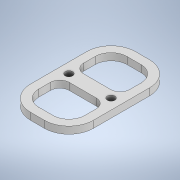
# Autodesk Inventor part: Top Seal 1
Saved by Autodesk Inventor 2021 (Build 250183000, 183)
## iProperties
Created: 2020-06-01
Part Number: Top Seal 1
Material: Generic
Document SubType Name: Modeling
Designer: jgray
Density: 1 g/cm^3
Appearance: Default
Author: jgray
Autodesk Inventor part; units mm, degrees
ref_plane "YZ Plane" through (0, 0, 0) normal (1, 0, 0) x (0, 1, 0)
ref_plane "XZ Plane" through (0, 0, 0) normal (0, 1, 0) x (-1, 0, 0)
ref_plane "XY Plane" through (0, 0, 0) normal (0, 0, 1) x (1, 0, 0)
sketch "Sketch2" plane through (0, 0, 0) normal (0, 1, 0) x (-1, 0, 0)
  arc A0 (3.5, 8.5) -> (1.5, 10.5) centre (1.5, 8.5) ccw
  arc A1 (1.5, -5.5) -> (3.5, -3.5) centre (1.5, -3.5) ccw
  line L0 (1.5, -5.5) -> (-1.5, -5.5)
  arc A2 (-3.5, -3.5) -> (-1.5, -5.5) centre (-1.5, -3.5) ccw
  arc A3 (-1.5, 10.5) -> (-3.5, 8.5) centre (-1.5, 8.5) ccw
  circle A4 centre (-9.4, -30.5) radius 1.7
  circle A5 centre (9.4, -15) radius 1.7
  circle A6 centre (9.4, 30.5) radius 1.7
  circle A7 centre (-9.4, 30.5) radius 1.7
  circle A8 centre (-9.4, 15) radius 1.7
  circle A9 centre (9.4, 15) radius 1.7
  circle A10 centre (-9.4, -15) radius 1.7
  circle A11 centre (9.4, -30.5) radius 1.7
  line L1 (-13.9, -33.875) -> (-13.9, 33.875)
  line L2 (13.9, -33.875) -> (-13.9, -33.875)
  line L3 (13.9, 33.875) -> (13.9, -33.875)
  line L4 (-13.9, 33.875) -> (13.9, 33.875)
  arc A12 (4.5, 8.5) -> (3.8682, 10.3417) centre (1.5, 8.5) ccw
  line L5 (-1.5, 10.5) -> (1.5, 10.5)
  arc A13 (-4.5, -3.5) -> (-1.5, -6.5) centre (-1.5, -3.5) ccw
  line L6 (-1.5, -6.5) -> (1.5, -6.5)
  arc A14 (1.5, -6.5) -> (4.5, -3.5) centre (1.5, -3.5) ccw
  arc A15 (4.5, 8.5) -> (1.5, 11.5) centre (1.5, 8.5) ccw
  line L7 (1.5, 11.5) -> (-1.5, 11.5)
  arc A16 (-1.5, 11.5) -> (-4.5, 8.5) centre (-1.5, 8.5) ccw
  line L8 (-1.5, 14.1) -> (1.5, 14.1)
  arc A17 (7.1, 8.5) -> (1.5, 14.1) centre (1.5, 8.5) ccw
  line L9 (7.1, 8.5) -> (7.1, -3.5)
  arc A18 (1.5, -9.1) -> (7.1, -3.5) centre (1.5, -3.5) ccw
  line L10 (1.5, -9.1) -> (-1.5, -9.1)
  arc A19 (-7.1, -3.5) -> (-1.5, -9.1) centre (-1.5, -3.5) ccw
  line L11 (-7.1, -3.5) -> (-7.1, 8.5)
  arc A20 (-1.5, 14.1) -> (-7.1, 8.5) centre (-1.5, 8.5) ccw
  line L12 (21.7007, 2.5) -> (-16.6227, 2.5) construction
  line L13 (4.9, 8.5) -> (4.9, 6.0503)
  arc A21 (1.5, -6.9) -> (4.9, -3.5) centre (1.5, -3.5) ccw
  line L14 (1.5, -6.9) -> (-1.5, -6.9)
  arc A22 (-4.9, -3.5) -> (-1.5, -6.9) centre (-1.5, -3.5) ccw
  line L15 (-4.9, 6.0503) -> (-4.9, 8.5)
  arc A23 (-1.5, 11.9) -> (-4.9, 8.5) centre (-1.5, 8.5) ccw
  line L16 (-1.5, 11.9) -> (1.5, 11.9)
  arc A24 (4.9, 8.5) -> (1.5, 11.9) centre (1.5, 8.5) ccw
  line L17 (6.7, -3.5) -> (6.7, 8.5)
  arc A25 (6.7, 8.5) -> (1.5, 13.7) centre (1.5, 8.5) ccw
  line L18 (1.5, 13.7) -> (-1.5, 13.7)
  arc A26 (-1.5, 13.7) -> (-6.7, 8.5) centre (-1.5, 8.5) ccw
  line L19 (-6.7, 8.5) -> (-6.7, -3.5)
  arc A27 (-6.7, -3.5) -> (-1.5, -8.7) centre (-1.5, -3.5) ccw
  line L20 (-1.5, -8.7) -> (1.5, -8.7)
  arc A28 (1.5, -8.7) -> (6.7, -3.5) centre (1.5, -3.5) ccw
  line L21 (2.9, 4.0503) -> (-2.9, 4.0503)
  line L22 (-2.9, 0.9497) -> (2.9, 0.9497)
  arc A29 (2.9, 4.0503) -> (4.9, 6.0503) centre (2.9, 6.0503) ccw
  arc A30 (-4.9, 6.0503) -> (-2.9, 4.0503) centre (-2.9, 6.0503) ccw
  line L23 (-4.9, -1.0503) -> (-4.9, -3.5)
  line L24 (4.9, -3.5) -> (4.9, -1.0503)
  arc A31 (4.9, -1.0503) -> (2.9, 0.9497) centre (2.9, -1.0503) ccw
  arc A32 (-2.9, 0.9497) -> (-4.9, -1.0503) centre (-2.9, -1.0503) ccw
  line L25 (-4.5, 8.5) -> (-4.5, 4.8503)
  line L26 (-4.5, 0.1497) -> (-4.5, -3.5)
  line L27 (-3.5, -3.5) -> (-3.5, 0.8576)
  line L28 (-3.5, 4.1424) -> (-3.5, 8.5)
  line L29 (3.5, 8.5) -> (3.5, 4.1424)
  line L30 (3.5, 0.8576) -> (3.5, -3.5)
  line L31 (4.5, -3.8243) -> (4.5, 0.1497)
  line L32 (4.5, 4.8503) -> (4.5, 8.5)
  line L33 (4.5, -3.5) -> (4.5, 0.1497)
  line L34 (4.5, 4.8503) -> (4.5, 8.5)
  circle A33 centre (-4.5, 2.5) radius 0.8
  circle A34 centre (4.5, 2.5) radius 0.8
  point P0 (0, 0)
  point P1 (0, 0)
  point P2 (2.621, 11.2827)
  point P3 (-2.6275, 11.2989)
  point P4 (3.8682, 10.3417)
  point P5 (4.5, 8.5)
  point P6 (4.5, -3.5)
  dimension "d10" = 2.6
  dimension "d11" = 23.2
  dimension "d12" = 14.2
  dimension "d15" = 23.2
  dimension "d17" = 0.4
  dimension "d18" = 2
  dimension "d19" = 2
  dimension "d20" = 1.6
  dimension "d21" = 1.6
  dimension "d22" = 2.2
  dimension "d23" = 2.2
  constraints: 70 end point, 60 point on circle, 35 centre point, 8 tangent, 4 point on line, 2 equal radius, 2 horizontal, 2 parallel, 1 vertical, 19 other
  measures "d10" distance between parallel lines of L7 L8
  measures "d11" distance between parallel lines of L10 L8
  measures "d12" distance between parallel lines of L11 L9
  measures "d15" diameter of L10 L12
  measures "d17" distance between parallel lines of L9 L17
  measures "d18" radius of A29
  measures "d19" radius of A31
  measures "d20" diameter of A33
  measures "d21" diameter of A34
  measures "d22" distance from line of L17 A34.centre
  measures "d23" distance from line of A33.centre L19
extrude "Extrusion1" add sketch "Sketch2" along normal blind 1.5 contours A28 L20 A27 L19 A26 L18 A25 L17
equation "\"d23\" = d22"
body "Solid1"
